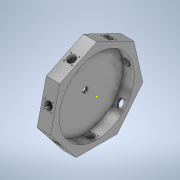
# Autodesk Inventor part: Peça14
Saved by Autodesk Inventor 2021 (Build 250183000, 183)
## iProperties
Created: 2021-07-17
Part Number: Peça14
Material: Aço
Document SubType Name: Modeling
Designer: Giovanni
Density: 7.85 g/cm^3
Appearance: Cromado - Preto polido
Author: Giovanni
Autodesk Inventor part; units mm, degrees
ref_plane "YZ Plane" through (0, 0, 0) normal (1, 0, 0) x (0, 1, 0)
ref_plane "XZ Plane" through (0, 0, 0) normal (0, 1, 0) x (-1, 0, 0)
ref_plane "XY Plane" through (0, 0, 0) normal (0, 0, 1) x (1, 0, 0)
sketch "Esboço1" plane through (0, 0, 0) normal (1, 0, 0) x (0, 1, 0)
  line L0 (599.9994, -0.8206) -> (373.452, -469.6101)
  line L1 (373.452, -469.6101) -> (-134.3125, -584.7736)
  line L2 (-134.3125, -584.7736) -> (-540.9369, -259.5907)
  line L3 (-540.9369, -259.5907) -> (-540.2248, 261.0693)
  line L4 (-540.2248, 261.0693) -> (-132.7124, 585.1388)
  line L5 (-132.7124, 585.1388) -> (374.7351, 468.5868)
  line L6 (374.7351, 468.5868) -> (599.9994, -0.8206)
  point P0 (0, 0)
  dimension "d44" = 600
  dimension "d45" = 520.66
  constraints: 14 end point, 15 other
  measures "d44" distance of L1.end point (0, 0)
  measures "d45" distance of L2.end L3.end
extrude "Extrusão1" add sketch "Esboço1" along normal blind 170
sketch "Esboço2" plane through (170, 0, 0) normal (1, 0, 0) x (0, 0, -1)
  circle A0 centre (0, 0) radius 475
  dimension "d11" = 950
  constraints: 1 centre point, 1 coincident
  measures "d11" diameter of A0
extrude "Extrusão2" cut sketch "Esboço2" against normal blind 146
sketch "Esboço3" plane through (0, -540.2248, 261.0693) normal (0, -0.6224199, 0.7826835) x (1, 0, 0)
  line L0 (0, 260.3302) -> (170, 260.3302) projected
  circle A0 centre (85, 260.3302) radius 50
  line L1 (170, 520.6605) -> (170, 0) projected
  line L2 (0, 520.6605) -> (0, 0) projected
  dimension "d14" = 100
  dimension "d15" = 85
  dimension "d53" = 170
  constraints: 1 centre point, 1 midpoint
  measures "d14" diameter of A0
  measures "d15" distance from line of L1 A0.centre
  measures "d53" distance between parallel lines of L1 L2
extrude "Extrusão3" cut sketch "Esboço3" against normal blind 95
sketch "Esboço5" plane through (0, -540.2248, 261.0693) normal (0, -0.6224199, 0.7826835) x (1, 0, 0)
  circle A0 centre (85, 260.3302) radius 50 projected
  point P0 (0, 260.3302)
  point P1 (35, 210.3302)
  point P2 (135, 210.3302)
  point P3 (135, 310.3302)
  point P4 (35, 310.3302)
  dimension "d54" = 50
  dimension "d55" = 50
  dimension "d56" = 50
  dimension "d57" = 50
  dimension "d62" = 50
  dimension "d63" = 50
  dimension "d64" = 50
  dimension "d65" = 50
  constraints: 1 coincident
  measures "d54" horizontal distance of point (85, 260.33) point (135, 310.33)
  measures "d55" horizontal distance of point (135, 210.33) point (85, 260.33)
  measures "d56" horizontal distance of point (85, 260.33) point (135, 210.33)
  measures "d57" horizontal distance of point (35, 210.33) point (85, 260.33)
  measures "d62" horizontal distance of point (85, 260.33) point (35, 210.33)
  measures "d63" horizontal distance of point (35, 310.33) point (85, 260.33)
  measures "d64" horizontal distance of point (85, 260.33) point (35, 310.33)
  measures "d65" horizontal distance of point (135, 310.33) point (85, 260.33)
hole "Furo1" at (135, -297.3344, 454.2251) at (135, -375.6028, 391.9831) at (35, -375.6028, 391.9831) at (35, -297.3344, 454.2251) direction (0, 0.6224199, -0.7826835) diameter 14.376 depth 95 tip angle 118 thread size "M16x1.5" class "6H" standard "ANSI Metric M Profile"
pattern_circular "Padrão circular1" count 7 over 360 about axis through (170, 0, 0) along (-1, 0, 0) of "Extrusão3", "Furo1"
sketch "Esboço6" plane through (24, 0, 0) normal (1, 0, 0) x (0, 0, -1)
  circle A0 centre (0, 0) radius 34
  dimension "d38" = 68
  constraints: 1 centre point, 1 coincident
  measures "d38" diameter of A0
extrude "Extrusão4" cut sketch "Esboço6" against normal blind 15
sketch "Esboço7" plane through (9, 0, 0) normal (1, 0, 0) x (0, 0, -1)
  circle A0 centre (0, 0) radius 27.5
  dimension "d41" = 55
  constraints: 1 centre point, 1 coincident
  measures "d41" diameter of A0
extrude "Extrusão5" cut sketch "Esboço7" against normal through all
sketch "Esboço9" plane through (170, 0, 0) normal (1, 0, 0) x (0, 0, -1)
  point P0 (0, 0)
